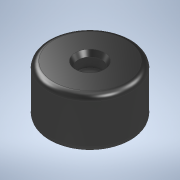
# Autodesk Inventor part: Motor
Saved by Autodesk Inventor 2021 (Build 250183000, 183)
## iProperties
Created: 2020-07-16
Part Number: Motor
Material: Generic
Document SubType Name: Modeling
Designer: Andrew
Density: 1 g/cm^3
Appearance: Default
Author: Andrew
Autodesk Inventor part; units mm, degrees
ref_plane "YZ Plane" through (0, 0, 0) normal (1, 0, 0) x (0, 1, 0)
ref_plane "XZ Plane" through (0, 0, 0) normal (0, 1, 0) x (-1, 0, 0)
ref_plane "XY Plane" through (0, 0, 0) normal (0, 0, 1) x (1, 0, 0)
sketch "Sketch1" plane through (0, 0, 0) normal (0, 1, 0) x (-1, 0, 0)
  circle A0 centre (0, 0) radius 15
  dimension "d0" = 30
  constraints: 1 centre point, 1 coincident
  measures "d0" diameter of A0
extrude "Extrusion1" add sketch "Sketch1" along normal blind 18
fillet "Fillet1" radius 2 2 edges at (15, 18, 0) (15, 0, 0)
sketch "Sketch4" plane through (0, 0, 0) normal (0, -1, 0) x (1, 0, 0)
  circle A0 centre (0, 0) radius 9.5 construction
  point P0 (0, 9.5)
  point P1 (0, -9.5)
  point P2 (-9.5, 0)
  point P3 (9.5, 0)
  dimension "d16" = 19
  constraints: 4 point on circle, 1 centre point, 1 coincident
  measures "d16" diameter of A0
hole "Hole1" at (0, 0, 9.5) at (0, 0, -9.5) at (-9.5, 0, 0) at (9.5, 0, 0) direction (0, 1, 0) diameter 3.242 depth 8 tip angle 118 thread size "M4x0.7" class "6H" standard "ISO Metric profile"
sketch "Sketch6" plane through (0, 18, 0) normal (0, 1, 0) x (1, 0, 0)
  line L0 (-3, 3) -> (3, 3) construction
  line L1 (3, 3) -> (3, -3) construction
  line L2 (3, -3) -> (-3, -3) construction
  line L3 (-3, -3) -> (-3, 3) construction
  circle A0 centre (0, 0) radius 4.2426
  dimension "d30" = 6
  dimension "d31" = 6
  dimension "d32" = 3
  dimension "d33" = 3
  constraints: 8 end point, 2 parallel, 1 coincident, 1 horizontal, 1 perpendicular, 3 other
  measures "d30" distance of L1.end L2.end
  measures "d31" distance of L0.end L1.end
  measures "d32" distance from line of point (0, 0) L1
  measures "d33" distance from line of point (0, 0) L0
extrude "Extrusion6" cut sketch "Sketch6" against normal blind 5
chamfer "Chamfer1" distance 1 angle 60 1 edges at (-4.2426, 18, 0) measured on face at (-9.9139, 18, -1.3755)
body "Solid1"
